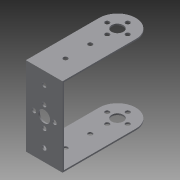
# Autodesk Inventor part: modelo 1
Saved by Autodesk Inventor 2014 (Build 180170000, 170)
## iProperties
Created: 2014-11-19
Part Number: modelo 1
Material: Generic
Document SubType Name: Modeling
Designer: alumnoutec
Density: 1 g/cm^3
Appearance: Default
Author: alumnoutec
Autodesk Inventor part; units mm, degrees
ref_plane "YZ Plane" through (0, 0, 0) normal (1, 0, 0) x (0, 1, 0)
ref_plane "XZ Plane" through (0, 0, 0) normal (0, 1, 0) x (-1, 0, 0)
ref_plane "XY Plane" through (0, 0, 0) normal (0, 0, 1) x (1, 0, 0)
sketch "Sketch1" plane through (0, 0, 0) normal (0, 0, 1) x (1, 0, 0)
  line L0 (-9.2684, -9.4429) -> (15.7316, -9.4429)
  line L1 (15.7316, -9.4429) -> (15.7316, 40.5571)
  arc A0 (15.7316, 40.5571) -> (-9.2684, 40.5571) centre (3.2316, 40.5571) ccw
  line L2 (-9.2684, 40.5571) -> (-9.2684, -9.4429)
  circle A1 centre (3.2316, 40.5571) radius 4
  circle A2 centre (-3.7684, 40.5571) radius 1.5
  circle A3 centre (3.2316, 47.5571) radius 1.5
  circle A4 centre (3.2316, 33.5571) radius 1.5
  circle A5 centre (10.2316, 40.5571) radius 1.5
  circle A6 centre (3.2316, 21.9571) radius 1.5
  circle A7 centre (3.2316, 5.0871) radius 1.5
  point P0 (0, 0)
  dimension "d0" = 25
  dimension "d1" = 50
  dimension "d3" = 8
  dimension "d5" = 3
  dimension "d6" = 3
  dimension "d7" = 3
  dimension "d8" = 3
  dimension "d10" = 3
  dimension "d12" = 3
  constraints: 8 centre point, 6 end point, 2 point on circle, 1 coincident, 1 horizontal, 1 perpendicular, 1 tangent
  measures "d0" distance of L0.start L0.end
  measures "d1" distance of L0.end L1.end
  measures "d3" diameter of A1
  measures "d5" diameter of A2
  measures "d6" diameter of A3
  measures "d7" diameter of A4
  measures "d8" diameter of A5
  measures "d10" diameter of A6
  measures "d12" diameter of A7
extrude "Extrusion1" add sketch "Sketch1" along normal blind 54
sketch "Sketch2" plane through (15.7316, -9.4429, 0) normal (1, 0, 0) x (0, 0, -1)
  line L0 (-54, 0) -> (-54, 50) projected
  line L1 (-54, 0) -> (-53, 0)
  line L2 (-53, 0) -> (-53, 1)
  line L3 (-53, 1) -> (-54, 1)
  line L4 (-54, 1) -> (-54, 0)
  line L5 (0, 0) -> (-1, 0)
  line L6 (-1, 0) -> (-1, 1)
  line L7 (-1, 1) -> (0, 1)
  line L8 (0, 1) -> (0, 0)
  line L9 (-53, 1) -> (-53, 62.5)
  line L10 (-53, 1) -> (-1, 1)
  line L11 (-1, 1) -> (-1, 62.5)
  line L12 (0, 50) -> (0, 50) projected
  line L13 (0, 50) -> (-54, 50) projected
  line L14 (-54, 50) -> (-54, 50) projected
  line L15 (0, 50) -> (-54, 50) projected
  line L16 (0, 62.5) -> (-54, 62.5) projected
  line L17 (-54, 62.5) -> (-54, 50) projected
  line L18 (0, 62.5) -> (0, 50) projected
  line L19 (0, 62.5) -> (-1, 62.5)
  line L20 (-1, 62.5) -> (-1, 0)
  line L21 (-1, 0) -> (0, 0)
  line L22 (0, 0) -> (0, 62.5)
  line L23 (-54, 62.5) -> (-53, 62.5)
  line L24 (-53, 62.5) -> (-53, 0)
  line L25 (-53, 0) -> (-54, 0)
  line L26 (-54, 0) -> (-54, 62.5)
  line L27 (-53, 62.5) -> (-1, 62.5)
  line L28 (-1, 62.5) -> (-1, 1)
  line L29 (-1, 1) -> (-53, 1)
  line L30 (-53, 1) -> (-53, 62.5)
  point P0 (0, 9.4429)
  dimension "d15" = 1
  dimension "d16" = 1
  dimension "d17" = 1
  dimension "d18" = 1
  constraints: 46 end point, 11 parallel, 6 perpendicular, 5 horizontal, 2 point on line
  measures "d15" distance of L3.end L2.end
  measures "d16" distance of L2.end L1.end
  measures "d17" distance of L6.end L7.end
  measures "d18" distance of L5.end L6.end
extrude "Extrusion2" cut sketch "Sketch2" against normal through all contours L9 L13 L11 L10 | L9 L16 L11 L13
sketch "Sketch3" plane through (15.7316, -8.4429, 53) normal (0, 1, 0) x (1, 0, 0)
  circle A0 centre (-12.5, 26) radius 4
  circle A1 centre (-12.5, 33) radius 1.5
  circle A2 centre (-19.5, 26) radius 1.5
  circle A3 centre (-12.5, 19) radius 1.5
  circle A4 centre (-5.5, 26) radius 1.5
  circle A5 centre (-12.5, 44.6) radius 1.5
  circle A6 centre (-12.5, 7.4) radius 1.5
  point P0 (-15.7316, 53)
  dimension "d23" = 3
  dimension "d26" = 360
  dimension "d29" = 3
  constraints: 7 centre point, 9 other
  measures "d23" diameter of A1
  measures "d29" diameter of A5
extrude "Extrusion3" cut sketch "Sketch3" against normal blind 58
body "Solid1"
